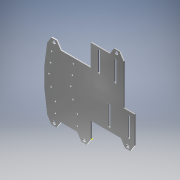
# Autodesk Inventor part: base_plate
Saved by Autodesk Inventor 2018 (Build 220112000, 112)
## iProperties
Created: 2018-04-04
Part Number: base_plate
Material: アルミニウム 6061
Document SubType Name: モデリング
Designer: NaMACHAN
Density: 2.7 g/cm^3
Appearance: アルミニウム - フラット
Sheet Metal Rule: Default
Mass: 92.2429 g
Surface Area: 369.048 cm^2
Volume: 34.164 cm^3
Author: NaMACHAN
Autodesk Inventor part; units mm, degrees
ref_plane "YZ Plane" through (0, 0, 0) normal (1, 0, 0) x (0, 1, 0)
ref_plane "XZ Plane" through (0, 0, 0) normal (0, 1, 0) x (-1, 0, 0)
ref_plane "XY Plane" through (0, 0, 0) normal (0, 0, 1) x (1, 0, 0)
sketch "スケッチ1" plane through (0, 0, 0) normal (0, 1, 0) x (-1, 0, 0)
  line L0 (80, 0) -> (85, 38)
  line L1 (85, 38) -> (85, 76)
  line L2 (85, 76) -> (80, 114)
  line L3 (-60, 80) -> (-60, 154)
  line L4 (0, 0) -> (0, 30)
  line L5 (-80, 30) -> (-80, 80)
  line L6 (-80, 80) -> (-60, 80)
  line L7 (0, 114) -> (0, 154)
  line L8 (-35, 154) -> (0, 154)
  line L9 (-52.5, 166) -> (-42.5, 166)
  line L10 (-42.5, 166) -> (-35, 154)
  line L11 (72.5, 126) -> (62.5, 126)
  line L12 (0, 114) -> (55, 114)
  line L13 (55, 114) -> (62.5, 126)
  line L14 (80, 114) -> (72.5, 126)
  line L15 (-52.5, 166) -> (-60, 154)
  line L16 (80, 0) -> (72.5, -12)
  line L17 (72.5, -12) -> (62.5, -12)
  line L18 (62.5, -12) -> (55, 0)
  line L19 (55, 0) -> (25, 0)
  line L20 (25, 0) -> (17.5, -12)
  line L21 (17.5, -12) -> (7.5, -12)
  line L22 (7.5, -12) -> (0, 0)
  line L23 (0, 30) -> (-55, 30)
  line L24 (-55, 30) -> (-62.5, 18)
  line L25 (-62.5, 18) -> (-72.5, 18)
  line L26 (-72.5, 18) -> (-80, 30)
  dimension "d4" = 38
  dimension "d6" = 5
  dimension "d29" = 80
  dimension "d34" = 38
  dimension "d128" = 38
  dimension "d182" = 30
  dimension "d186" = 50
  dimension "d190" = 40
  dimension "d204" = 80
  dimension "d218" = 35
  dimension "d219" = 20
  dimension "d222" = 10
  dimension "d224" = 10
  dimension "d225" = 55
  dimension "d226" = 80
  dimension "d227" = 7.5
  dimension "d228" = 12
  dimension "d229" = 60
  dimension "d230" = 7.5
  dimension "d231" = 12
  dimension "d232" = 30
  dimension "d233" = 10
  dimension "d234" = 10
  dimension "d235" = 7.5
  dimension "d236" = 7.5
  dimension "d237" = 12
  dimension "d238" = 7.5
  dimension "d239" = 55
  dimension "d240" = 10
  dimension "d241" = 7.5
  dimension "d242" = 12
  constraints: 55 end point, 6 horizontal, 6 horizontal alignment, 3 parallel, 3 perpendicular, 2 vertical, 2 vertical alignment, 1 coincident
  measures "d4" vertical distance of L0.start L0.end
  measures "d6" horizontal distance of L0.start L0.end
  measures "d29" distance of L4.start L0.start
  measures "d34" vertical distance of L2.end L1.end
  measures "d128" distance of L0.end L1.end
  measures "d182" distance of L4.start L4.end
  measures "d186" distance of L5.start L5.end
  measures "d190" distance of L7.start L7.end
  measures "d204" distance of L4.end L5.start
  measures "d218" distance of L8.start L7.end
  measures "d219" distance of L5.end L3.start
  measures "d222" distance of L9.start L9.end
  measures "d224" distance of L11.start L11.end
  measures "d225" distance of L7.start L12.end
  measures "d226" distance of L2.end L7.start
  measures "d227" horizontal distance of L11.end L12.end
  measures "d228" vertical distance of L11.start L2.end
  measures "d229" distance of L3.end L7.end
  measures "d230" horizontal distance of L3.end L9.start
  measures "d231" vertical distance of L9.start L3.end
  measures "d232" distance of L18.end L19.end
  measures "d233" distance of L16.end L17.end
  measures "d234" distance of L20.end L21.end
  measures "d235" horizontal distance of L0.start L16.end
  measures "d236" horizontal distance of point (0, 0) L21.end
  measures "d237" distance between parallel lines of L19 L17
  measures "d238" horizontal distance of L18.end L17.end
  measures "d239" distance of L4.end L23.end
  measures "d240" distance of L24.end L25.end
  measures "d241" horizontal distance of L24.end L23.end
  measures "d242" distance from line of L5.start L25
extrude "押し出し1" add sketch "スケッチ1" along normal blind 2
fillet "フィレット1" radius 2 4 edges at (52.5, 1, 166) (-80, 1, 114) (0, 1, 0) (-80, 1, 0)
sketch "スケッチ8" plane through (0, 2, 0) normal (0, 1, 0) x (1, 0, 0)
  point P0 (0, 0)
  point P1 (-65, -9.5)
  point P2 (-25, -9.5)
  point P3 (-25, -28.5)
  point P4 (-65, -28.5)
  point P5 (-73, -47.5)
  point P6 (-33, -47.5)
  point P7 (-77, -66.5)
  point P8 (-37, -66.5)
  point P9 (-34, -85.5)
  point P10 (-74, -85.5)
  point P11 (-72, -104.5)
  point P12 (-32, -104.5)
  dimension "d132" = 40
  dimension "d133" = 40
  dimension "d134" = 40
  dimension "d135" = 40
  dimension "d136" = 40
  dimension "d137" = 40
  dimension "d138" = 9.5
  dimension "d139" = 25
  dimension "d141" = 19
  dimension "d143" = 19
  dimension "d144" = 19
  dimension "d145" = 19
  dimension "d146" = 19
  dimension "d147" = 8
  dimension "d148" = 4
  dimension "d149" = 3
  dimension "d150" = 2
  constraints: 6 horizontal alignment, 1 vertical alignment
  measures "d132" distance of point (-25, -9.5) point (-65, -9.5)
  measures "d133" distance of point (-65, -28.5) point (-25, -28.5)
  measures "d134" distance of point (-73, -47.5) point (-33, -47.5)
  measures "d135" distance of point (-77, -66.5) point (-37, -66.5)
  measures "d136" distance of point (-34, -85.5) point (-74, -85.5)
  measures "d137" distance of point (-32, -104.5) point (-72, -104.5)
  measures "d138" vertical distance of point (0, 0) point (-25, -9.5)
  measures "d139" horizontal distance of point (0, 0) point (-25, -9.5)
  measures "d141" distance of point (-25, -28.5) point (-25, -9.5)
  measures "d143" vertical distance of point (-33, -47.5) point (-25, -28.5)
  measures "d144" vertical distance of point (-37, -66.5) point (-33, -47.5)
  measures "d145" vertical distance of point (-34, -85.5) point (-37, -66.5)
  measures "d146" vertical distance of point (-32, -104.5) point (-34, -85.5)
  measures "d147" horizontal distance of point (-25, -28.5) point (-33, -47.5)
  measures "d148" horizontal distance of point (-37, -66.5) point (-33, -47.5)
  measures "d149" horizontal distance of point (-34, -85.5) point (-37, -66.5)
  measures "d150" horizontal distance of point (-34, -85.5) point (-32, -104.5)
hole "穴6" at (-65, 2, 9.5) at (-25, 2, 9.5) at (-25, 2, 28.5) at (-65, 2, 28.5) at (-73, 2, 47.5) at (-33, 2, 47.5) at (-77, 2, 66.5) at (-37, 2, 66.5) at (-34, 2, 85.5) at (-74, 2, 85.5) at (-72, 2, 104.5) at (-32, 2, 104.5) direction (0, -1, 0) diameter 3 end through all
sketch "スケッチ11" plane through (0, 2, 0) normal (0, 1, 0) x (1, 0, 0)
  line L0 (47, -114) -> (47, -149)
  arc A0 (43, -149) -> (47, -149) centre (45, -149) ccw
  line L1 (43, -149) -> (43, -114)
  arc A1 (47, -114) -> (43, -114) centre (45, -114) ccw
  line L2 (17, -114) -> (17, -149)
  arc A2 (13, -149) -> (17, -149) centre (15, -149) ccw
  line L3 (13, -149) -> (13, -114)
  arc A3 (17, -114) -> (13, -114) centre (15, -114) ccw
  line L4 (0, -154) -> (35, -154) projected
  line L5 (0, -114) -> (0, -154) projected
  point P0 (0, 0)
  point P1 (50, -163)
  dimension "d194" = 2
  dimension "d198" = 2
  dimension "d199" = 30
  dimension "d220" = 5
  dimension "d221" = 40
  dimension "d256" = 15
  constraints: 8 end point, 8 point on circle, 8 tangent, 4 centre point, 2 horizontal alignment, 2 parallel, 2 vertical
  measures "d194" radius of A1
  measures "d198" radius of A2
  measures "d199" distance of A0.centre A2.centre
  measures "d220" distance from line of L4 A0.centre
  measures "d221" distance from line of A1.centre L4
  measures "d256" distance from line of L5 A2.centre
extrude "押し出し3" cut sketch "スケッチ11" against normal blind 10
sketch "スケッチ12" plane through (0, 2, 0) normal (0, 1, 0) x (1, 0, 0)
  point P0 (0, 0)
sketch "スケッチ13" plane through (0, 2, 0) normal (0, 1, 0) x (1, 0, 0)
  line L0 (68, -72) -> (68, -38)
  arc A0 (72, -38) -> (68, -38) centre (70, -38) ccw
  line L1 (72, -38) -> (72, -72)
  arc A1 (68, -72) -> (72, -72) centre (70, -72) ccw
  line L2 (36, -72) -> (36, -38)
  arc A2 (36, -38) -> (32, -38) centre (34, -38) ccw
  line L3 (32, -38) -> (32, -72)
  arc A3 (32, -72) -> (36, -72) centre (34, -72) ccw
  line L4 (80, -80) -> (80, -30) projected
  line L5 (60, -80) -> (80, -80) projected
  line L6 (55, -30) -> (0, -30) projected
  point P0 (0, 0)
  dimension "d205" = 2
  dimension "d206" = 2
  dimension "d207" = 10
  dimension "d208" = 8
  dimension "d210" = 36
  dimension "d243" = 8
  constraints: 8 end point, 8 point on circle, 8 tangent, 4 centre point, 2 horizontal alignment, 2 parallel, 2 vertical
  measures "d205" radius of A3
  measures "d206" radius of A1
  measures "d207" distance from line of L4 A1.centre
  measures "d208" distance from line of L5 A1.centre
  measures "d210" distance of A0.centre A2.centre
  measures "d243" distance from line of L6 A0.centre
extrude "押し出し4" cut sketch "スケッチ13" against normal blind 10
sketch "スケッチ14" plane through (0, 0, 0) normal (0, -1, 0) x (1, 0, 0)
  line L0 (-62.5, 126) -> (-72.5, 126) projected
  line L1 (-72.5, -12) -> (-62.5, -12) projected
  line L2 (-17.5, -12) -> (-7.5, -12) projected
  line L3 (62.5, 18) -> (72.5, 18) projected
  line L4 (51.3915, 166) -> (42.5, 166) projected
  point P0 (0, 0)
  point P1 (-67.5, -7)
  point P2 (-12.5, -7)
  point P3 (-67.5, 121)
  point P4 (67.5, 23)
  point P5 (46.9458, 161)
  point P6 (-67.5, 126)
  point P7 (-67.5, -12)
  point P8 (-12.5, -12)
  point P9 (67.5, 18)
  point P10 (46.9458, 166)
  dimension "d244" = 5
  dimension "d245" = 5
  dimension "d246" = 5
  dimension "d247" = 5
  dimension "d248" = 5
  constraints: 5 midpoint, 5 vertical alignment
  measures "d244" distance from line of point (46.946, 161) L4
  measures "d245" distance from line of point (-67.5, 121) L0
  measures "d246" distance from line of L1 point (-67.5, -7)
  measures "d247" distance of point (-12.5, -12) point (-12.5, -7)
  measures "d248" distance from line of L3 point (67.5, 23)
hole "穴9" at (46.9458, 0, 161) at (-67.5, 0, 121) at (-67.5, 0, -7) at (-12.5, 0, -7) at (67.5, 0, 23) direction (0, 1, 0) diameter 6 end through all
sketch "スケッチ16" plane through (0, 2, 0) normal (0, 1, 0) x (1, 0, 0)
  line L0 (-7.0834, -94.7024) -> (16.1275, -54.5)
  arc A0 (16.1275, -54.5) -> (13.5294, -50) centre (13.5294, -53) ccw
  line L1 (13.5294, -50) -> (-20, -50)
  arc A1 (-20, -50) -> (-22.5981, -54.5) centre (-20, -53) ccw
  line L2 (-22.5981, -54.5) -> (-12.9166, -94.7024)
  arc A2 (-12.9166, -94.7024) -> (-7.0834, -94.7024) centre (-10, -94) ccw
  line L3 (55, -30) -> (0, -30) projected
  line L4 (-55, -114) -> (0, -114) projected
  point P0 (0, 0)
  dimension "d264" = 20
  dimension "d265" = 20
  dimension "d266" = 20
  dimension "d267" = 3
  dimension "d268" = 3
  dimension "d269" = 3
  dimension "d270" = 120
  dimension "d271" = 120
  dimension "d272" = 10
  constraints: 6 end point, 6 point on circle, 4 tangent, 3 centre point, 1 horizontal, 1 horizontal alignment
  measures "d264" distance between parallel lines of L3 L1
  measures "d265" distance from line of L4 A2.centre
  measures "d266" horizontal distance of A1.centre L3.end
  measures "d267" radius of A1
  measures "d268" radius of A0
  measures "d269" radius of A2
  measures "d272" horizontal distance of L4.end A2.centre
extrude "押し出し6" cut sketch "スケッチ16" against normal blind 10
